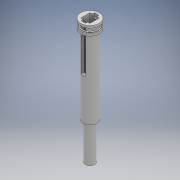
# Autodesk Inventor part: Handle
Saved by Autodesk Inventor 2018 (Build 220112000, 112)
## iProperties
Created: 2019-07-18
Part Number: Handle
Material: Generic
Document SubType Name: Modeling
Designer: aal_9
Density: 1 g/cm^3
Appearance: Default
Author: aal_9
Autodesk Inventor part; units mm, degrees
ref_plane "YZ Plane" through (0, 0, 0) normal (1, 0, 0) x (0, 1, 0)
ref_plane "XY Plane" through (0, 0, 0) normal (0, 0, 1) x (1, 0, 0)
sketch "Sketch1" plane through (0, 0, 0) normal (0, 0, 1) x (1, 0, 0)
  circle A0 centre (0, 0) radius 5
  dimension "d0" = 10
  constraints: 1 centre point, 1 coincident
  measures "d0" diameter of A0
extrude "Extrusion1" add sketch "Sketch1" along normal blind 40
sketch "Sketch3" plane through (0, 0, 40) normal (0, 0, 1) x (1, 0, 0)
  circle A0 centre (0, 0) radius 7.5
  dimension "d13" = 15
  constraints: 1 centre point, 1 coincident
  measures "d13" diameter of A0
extrude "Extrusion3" add sketch "Sketch3" along normal blind 95
sketch "Sketch4" plane through (0, 0, 135) normal (0, 0, 1) x (1, 0, 0)
  circle A0 centre (0, 0) radius 4.45
  dimension "d16" = 8.9
  constraints: 1 centre point, 1 coincident
  measures "d16" diameter of A0
extrude "Extrusion4" cut sketch "Sketch4" against normal blind 55
ref_plane "Work Plane2" through (0, 7.5, 40) normal (0, 1, 0) x (-1, 0, 0)
sketch "Sketch5" plane through (0, 7.5, 40) normal (0, 1, 0) x (-1, 0, 0)
  line L0 (2.5, 95) -> (-2.5, 95)
  line L1 (-2.5, 95) -> (-2.5, 45)
  line L2 (-2.5, 45) -> (2.5, 45)
  line L3 (2.5, 45) -> (2.5, 95)
  line L4 (7.5, 95) -> (-7.5, 95) projected
  point P0 (0, -40)
  dimension "d19" = 0
  dimension "d20" = 5
  dimension "d21" = 2.5
  dimension "d22" = 50
  constraints: 8 end point, 2 parallel, 1 horizontal, 1 perpendicular
  measures "d19" distance between parallel lines of L0 L4
  measures "d20" distance of L0.start L0.end
  measures "d21" distance from line of point (0, -40) L3
  measures "d22" distance of L2.end L0.start
extrude "Extrusion5" cut sketch "Sketch5" against normal through all
sketch "Sketch6" plane through (0, 0, 80) normal (0, 0, 1) x (1, 0, 0)
  circle A0 centre (0, 0) radius 3.2
  dimension "d25" = 6.4
  constraints: 1 centre point, 1 coincident
  measures "d25" diameter of A0
extrude "Extrusion6" cut sketch "Sketch6" against normal blind 35
sketch "Sketch7" plane through (0, 0, 135) normal (0, 0, 1) x (1, 0, 0)
  line L0 (-5, 5) -> (5, 5)
  line L1 (5, 5) -> (5, -5)
  line L2 (5, -5) -> (-5, -5)
  line L3 (-5, -5) -> (-5, 5)
  circle A0 centre (0, 0) radius 3.2 projected
  dimension "d29" = 10
  dimension "d30" = 10
  dimension "d31" = 5
  dimension "d32" = 5
  constraints: 8 end point, 2 parallel, 1 horizontal, 1 perpendicular
  measures "d29" distance of L1.end L2.end
  measures "d30" distance of L0.end L1.end
  measures "d31" distance from line of A0.centre L0
  measures "d32" distance from line of A0.centre L1
extrude "Extrusion7" cut sketch "Sketch7" against normal blind 10
sketch "Sketch9" plane through (0, 0, 135) normal (0, 0, 1) x (1, 0, 0)
  circle A0 centre (0, 0) radius 10
  circle A1 centre (0, 0) radius 7.5
  dimension "d39" = 20
  dimension "d42" = 15
  constraints: 2 centre point, 2 coincident
  measures "d39" diameter of A0
  measures "d42" diameter of A1
extrude "Extrusion8" add sketch "Sketch9" against normal blind 10
sketch "Sketch10" plane through (0, 0, 0) normal (1, 0, 0) x (0, 1, 0)
  line L0 (7.5, 132) -> (10, 132)
  line L1 (10, 132) -> (10, 128)
  line L2 (10, 128) -> (7.5, 128)
  line L3 (7.5, 128) -> (7.5, 132)
  line L4 (-10, 125) -> (10, 125) projected
  line L5 (0, -27) -> (0, 162) projected
  line L6 (10, 135) -> (10, 125) projected
  line L7 (9, 127.5) -> (10, 127.5)
  line L8 (10, 127.5) -> (10, 132.5)
  line L9 (10, 132.5) -> (9, 132.5)
  line L10 (9, 132.5) -> (9, 127.5)
  line L11 (-10, 135) -> (10, 135) projected
  point P0 (0, 0)
  dimension "d43" = 4
  dimension "d44" = 3
  dimension "d46" = 2.5
  dimension "d47" = 10
  dimension "d49" = 5
  dimension "d50" = 2.5
  dimension "d51" = 1
  constraints: 16 end point, 4 parallel, 2 horizontal, 2 perpendicular, 1 point on line
  measures "d43" distance of L2.end L0.start
  measures "d44" distance between parallel lines of L4 L2
  measures "d46" distance of L0.start L0.end
  measures "d47" distance from line of point (0, 0) L1
  measures "d49" distance of L9.end L7.start
  measures "d50" distance between parallel lines of L11 L9
  measures "d51" distance of L7.start L7.end
revolve "Revolution1" cut sketch "Sketch10" angle 360 about axis through (0, 0, -10) along (0, 0, 1) contours L0 L10 L2 L3 | L10 L9 L6 L0 | L0 L1 L2 L10 | L2 L6 L7 L10
ref_plane "Work Plane3" through (0, 10, 135) normal (0, 1, 0) x (-1, 0, 0)
equation "\"d21\" = 0.5 * d20"
equation "\"d31\" = 0.5 * d30"
equation "\"d32\" = 0.5 * d29"
body "Solid1"
